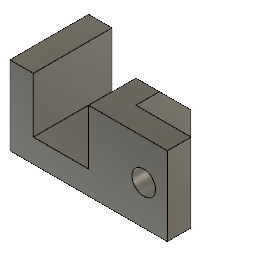
class4example v4 (Autodesk Fusion 360 design; units mm, degrees)
Autodesk Fusion 360 part; units mm, degrees
sketch "Sketch1" plane through (0, 0, 0) normal (0, 0, 1) x (1, 0, 0) in component "Component"
  line L0 (0, 0) -> (63.5, 0)
  line L1 (63.5, 0) -> (63.5, 19.05)
  line L2 (63.5, 19.05) -> (19.05, 19.05)
  line L3 (19.05, 19.05) -> (19.05, 63.5)
  line L4 (19.05, 63.5) -> (0, 63.5)
  line L5 (0, 63.5) -> (0, 0)
  dimension "d1" = 63.5
  dimension "d2" = 63.5
  dimension "d3" = 19.05
  dimension "d4" = 19.05
  measures "d2" distance of L0.start
  measures "d3" distance of L0.start
extrude "Extrude1" add sketch "Sketch1" along normal blind 63.5 in component "Component"
sketch "Sketch2" plane through (0, 63.5, 0) normal (0, 1, 0) x (-1, 0, 0) in component "Component"
  line L0 (-19.05, 0) -> (0, 0)
  line L1 (0, 0) -> (0, 63.5)
  line L2 (0, 63.5) -> (-19.05, 63.5)
  line L3 (-19.05, 63.5) -> (-19.05, 0)
  line L4 (0, 0) -> (63.5, 0)
  line L5 (63.5, 0) -> (63.5, 63.5)
  line L6 (63.5, 63.5) -> (44.45, 63.5)
  line L7 (44.45, 63.5) -> (44.45, 19.05)
  line L8 (44.45, 19.05) -> (0, 19.05)
  line L9 (0, 19.05) -> (0, 0)
  dimension "d7" = 63.5
  dimension "d8" = 63.5
  dimension "d9" = 19.05
  dimension "d10" = 19.05
  measures "d9" distance of L0.end
extrude "Extrude2" add sketch "Sketch2" against normal blind 63.5 contours L1 L4 L5 L6 L7 L8 L9 in component "Component"
sketch "Sketch3" plane through (0, 19.05, 0) normal (0, 1, 0) x (-1, 0, 0) in component "Component"
  line L0 (-63.5, 0) -> (-19.05, 0)
  line L1 (-19.05, 0) -> (-19.05, 63.5)
  line L2 (-19.05, 63.5) -> (-63.5, 63.5)
  line L3 (-63.5, 63.5) -> (-63.5, 0)
  circle A0 centre (-44.45, 31.75) radius 9.525
  dimension "d13" = 19.05
  dimension "d14" = 31.75
  dimension "d15" = 19.05
  measures "d13" diameter of A0
  measures "d14" distance of L0 origin
extrude "Extrude3" cut sketch "Sketch3" against normal through all contours A0 in component "Component"
sketch "Sketch4" plane through (19.05, 0, 0) normal (1, 0, 0) x (0, 1, 0) in component "Component"
  line L0 (19.05, 0) -> (63.5, 0)
  line L1 (63.5, 0) -> (63.5, 63.5)
  line L2 (63.5, 63.5) -> (19.05, 63.5)
  line L3 (19.05, 63.5) -> (19.05, 0)
  line L4 (63.5, 38.1) -> (38.1, 63.5)
  dimension "d17" = 25.4
  dimension "d18" = 45
  measures "d18" angle of L2 L4
extrude "Extrude4" cut sketch "Sketch4" against normal up to surface (19.05 mm away) contours L1 L2 L4 in component "Component"
component "Component" placed x (1, 0, 0) y (0, 1, 0) z (0, 0, 1) at (0, 0, 0)
